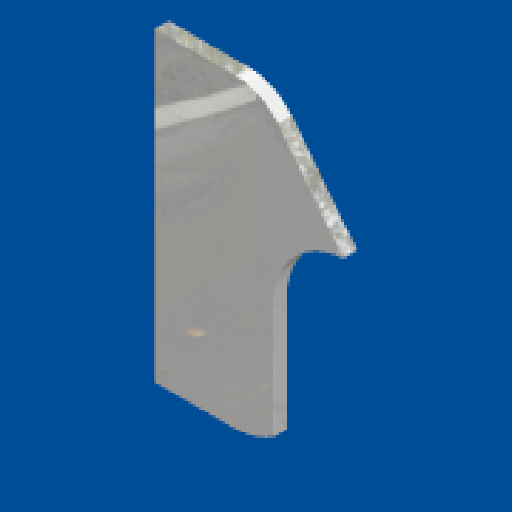
# Autodesk Inventor part: baseInner
Saved by Autodesk Inventor 2023 (Build 270158030, 158C)
## iProperties
Created: 2023-03-03
Part Number: baseInner
Material: Aluminum 6061
Document SubType Name: Modeling
Designer: kumpu
Density: 2.7 g/cm^3
Appearance: Aluminum - Dark
Mass: 151.363 g
Surface Area: 203.764 cm^2
Volume: 56.0605 cm^3
Author: kumpu
Autodesk Inventor part; units mm, degrees
ref_plane "YZ Plane" through (0, 0, 0) normal (1, 0, 0) x (0, 1, 0)
ref_plane "XZ Plane" through (0, 0, 0) normal (0, 1, 0) x (-1, 0, 0)
ref_plane "Work Plane1" through (0, 0, -12.7) normal (0, 0, 1) x (1, 0, 0)
sketch "Sketch1" plane through (0, 0, -12.7) normal (0, 0, 1) x (1, 0, 0)
  line L0 (-47.625, 69.85) -> (-11.1125, 69.85)
  arc A0 (8.9541, 60.0222) -> (-11.1125, 69.85) centre (-11.1125, 44.45) ccw
  line L1 (8.9541, 60.0222) -> (38.3789, 22.1047)
  line L2 (-47.625, 69.85) -> (-47.625, -69.85)
  line L3 (-47.625, -69.85) -> (-12.2749, -69.85)
  arc A1 (-12.2749, -69.85) -> (9.777, -62.1413) centre (-12.2749, -34.4543) ccw
  line L4 (9.777, -62.1413) -> (30.2464, -45.838)
  arc A2 (38.3789, 22.1047) -> (30.2464, -45.838) centre (41.275, -12.7) ccw
  line L5 (56.3249, -1.0209) -> (8.9541, 60.0222) construction
  line L6 (-11.1125, 69.85) -> (-60.325, 69.85) construction
  line L7 (-60.325, -69.85) -> (-12.2749, -69.85) construction
  line L8 (9.777, -62.1413) -> (53.1434, -27.6012) construction
  circle A3 centre (41.275, -12.7) radius 9.525 construction
  line L9 (-60.325, 69.85) -> (-60.325, -69.85) construction
  circle A4 centre (-11.1125, 44.45) radius 10
  line L10 (6.35, -12.7) -> (6.35, -64.8708)
  line L11 (41.275, 22.225) -> (38.2856, 22.225)
  point P0 (0, 0)
  point P1 (16.8552, -56.5037)
  point P2 (38.2856, 22.225)
  point P3 (6.35, -64.5536)
  dimension "d0" = 12.7
  dimension "d1" = 34.925
  dimension "d4" = 20
  constraints: 14 end point, 8 point on circle, 6 tangent, 4 centre point, 4 collinear, 2 perpendicular, 2 point on line, 1 coincident, 1 concentric, 1 horizontal, 1 parallel, 1 vertical
  measures "d0" distance between parallel lines of L9 L2
  measures "d1" radius of A2
  measures "d4" diameter of A4
extrude "Extrusion1" add sketch "Sketch1" along normal blind 6.35 contours L0 A0 L1 A2 L10 A1 L3 L2 | A4
body "Solid1"
